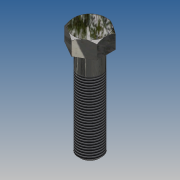
# Autodesk Inventor part: Sechskantenschraube_ra8846s
Saved by Autodesk Inventor 2021 (Build 250183000, 183)
## iProperties
Created: 2020-11-17
Part Number: Sechskantenschraube_ra8846s
Material: Stahl, hochfest, niedrig legiert
Document SubType Name: Modeling
Designer: Ricardo A
Density: 9.333 g/cm^3
Appearance: Stahl - poliert
Description: Motor_Teil7_6Schraube
Mass: 5 g
Surface Area: 4.73563 cm^2
Volume: 0.535733 cm^3
Author: Sander
Revision Number: Rev00
Autodesk Inventor part; units mm, degrees
ref_plane "YZ-Ebene" through (0, 0, 0) normal (1, 0, 0) x (0, 1, 0)
ref_plane "XZ-Ebene" through (0, 0, 0) normal (0, 1, 0) x (-1, 0, 0)
ref_plane "XY-Ebene" through (0, 0, 0) normal (0, 0, 1) x (1, 0, 0)
sketch "Skizze1" plane through (0, 0, 0) normal (0, 0, 1) x (1, 0, 0)
  line L0 (-4.8497, 0) -> (4.8497, 0) projected
  line L1 (0, -5.6) -> (0, 5.6) projected
  line L2 (0, 4) -> (3.4641, 2)
  line L3 (3.4641, 2) -> (3.4641, -2)
  line L4 (3.4641, -2) -> (0, -4)
  line L5 (0, -4) -> (-3.4641, -2)
  line L6 (-3.4641, -2) -> (-3.4641, 2)
  line L7 (-3.4641, 2) -> (0, 4)
  point P0 (0, 0)
  dimension "d9" = 8
  constraints: 12 end point, 2 midpoint, 1 point on line, 13 other
  measures "d9" distance of L2.start L4.end
extrude "Extrusion1" add sketch "Skizze1" along normal blind 3.5
sketch "Skizze2" plane through (0, 0, 3.5) normal (0, 0, 1) x (1, 0, 0)
  line L0 (3.4641, 2) -> (0, 4) projected
  circle A0 centre (0, 0) radius 3.4641
  constraints: 1 centre point, 1 coincident, 1 tangent
extrude "Extrusion2" cut sketch "Skizze2" against normal blind 3.5 draft 45 keep common part
sketch "Skizze3" plane through (0, 0, 0) normal (0, 0, -1) x (-1, 0, 0)
  circle A0 centre (0, 0) radius 2.5
  dimension "d6" = 5
  constraints: 1 centre point, 1 coincident
  measures "d6" diameter of A0
extrude "Extrusion3" add sketch "Skizze3" along normal blind 20
chamfer "Fase1" distance 0.5 angle 45 1 edges at (2.5, 0, -20)
thread "Gewinde1" size "M5x0.5" class "6g" standard "ISO Metric profile" length 15
thread "Gewinde2" size "M5x0.5" class "6g" standard "ISO Metric profile" length 15
thread "Gewinde3" size "M5x0.5" class "6g" standard "ISO Metric profile" length 15.5
